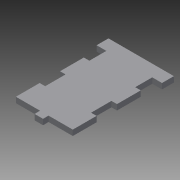
# Autodesk Inventor part: arm-servo
Saved by Autodesk Inventor 2013 (Build 170138000, 138)
## iProperties
Created: 2012-09-08
Part Number: arm-servo
Material: Generic
Document SubType Name: Modeling
Designer: frankenteddy
Density: 1 g/cm^3
Author: frankenteddy
Autodesk Inventor part; units mm, degrees
ref_plane "YZ Plane" through (0, 0, 0) normal (1, 0, 0) x (0, 1, 0)
ref_plane "XZ Plane" through (0, 0, 0) normal (0, 1, 0) x (-1, 0, 0)
ref_plane "XY Plane" through (0, 0, 0) normal (0, 0, 1) x (1, 0, 0)
sketch "Block1" plane through (0, 0, 0) normal (0, 0, 1) x (1, 0, 0)
  circle A0 centre (74.029, 24.2723) radius 1
  line L0 (49.279, 30.4723) -> (71.779, 30.4723)
  line L1 (71.779, 30.4723) -> (71.779, 18.0723)
  line L2 (71.779, 18.0723) -> (49.279, 18.0723)
  line L3 (49.279, 18.0723) -> (49.279, 30.4723)
  line L4 (49.279, 30.4723) -> (44.779, 30.4723)
  line L5 (44.779, 30.4723) -> (44.779, 18.0723)
  line L6 (44.779, 18.0723) -> (49.279, 18.0723)
  line L7 (49.279, 18.0723) -> (49.279, 30.4723)
  line L8 (71.779, 30.4723) -> (76.279, 30.4723)
  line L9 (76.279, 30.4723) -> (76.279, 18.0723)
  line L10 (76.279, 18.0723) -> (71.779, 18.0723)
  line L11 (71.779, 18.0723) -> (71.779, 30.4723)
  line L12 (44.779, 24.2723) -> (76.279, 24.2723) construction
  line L13 (47.029, 30.4723) -> (47.029, 18.0723) construction
  circle A1 centre (47.029, 24.2723) radius 1
  line L14 (74.029, 30.4723) -> (74.029, 18.0723) construction
  point P0 (60.979, 24.0984)
  dimension "d7" = 22.5
  dimension "d8" = 12.4
  dimension "d9" = 4.5
  dimension "d10" = 4.5
  dimension "d11" = 2
  dimension "d12" = 2
  measures "d7" distance of L1.end L2.end
  measures "d8" distance of L0.end L1.end
  measures "d9" distance of L6.end L5.end
  measures "d10" distance of L9.end L10.end
  measures "d11" diameter of A0
  measures "d12" diameter of A1
sketch "Sketch1" plane through (0, 0, 0) normal (0, 0, 1) x (1, 0, 0)
  line L0 (-38.4282, 40.714) -> (0.0718, 40.714)
  line L1 (0.0718, 40.714) -> (0.0718, 33.714)
  line L2 (0.0718, 33.714) -> (-38.4282, 33.714)
  line L3 (-38.4282, 33.714) -> (-38.4282, 40.714)
  line L4 (-92.7646, -8.503) -> (-89.7646, -8.503)
  line L5 (-89.7646, -8.503) -> (-89.7646, -11.753)
  line L6 (-89.7646, -11.753) -> (-92.7646, -11.753)
  line L7 (-92.7646, -11.753) -> (-92.7646, -8.503)
  line L8 (-92.7646, -21.6527) -> (-89.7646, -21.6527)
  line L9 (-89.7646, -21.6527) -> (-89.7646, -21.7527)
  line L10 (-89.7646, -21.7527) -> (-92.7646, -21.7527)
  line L11 (-92.7646, -21.7527) -> (-92.7646, -21.6527)
  line L12 (-32.6782, 33.714) -> (-5.6782, 33.714)
  line L13 (-5.6782, 33.714) -> (-5.6782, -16.286)
  line L14 (-5.6782, -16.286) -> (-32.6782, -16.286)
  line L15 (-32.6782, -16.286) -> (-32.6782, 33.714)
  line L16 (-19.1782, 40.714) -> (-19.1782, 33.714) construction
  line L17 (-19.1782, -16.286) -> (-19.1782, 33.714) construction
  line L18 (-35.9282, 23.714) -> (-32.6782, 23.714)
  line L19 (-32.6782, 23.714) -> (-32.6782, 9.714)
  line L20 (-32.6782, 9.714) -> (-35.9282, 9.714)
  line L21 (-35.9282, 9.714) -> (-35.9282, 23.714)
  line L22 (-2.4282, 23.714) -> (-5.6782, 23.714)
  line L23 (-5.6782, 23.714) -> (-5.6782, 9.714)
  line L24 (-5.6782, 9.714) -> (-2.4282, 9.714)
  line L25 (-2.4282, 9.714) -> (-2.4282, 23.714)
  line L26 (-35.9282, -2.286) -> (-32.6782, -2.286)
  line L27 (-32.6782, -2.286) -> (-32.6782, -16.286)
  line L28 (-32.6782, -16.286) -> (-35.9282, -16.286)
  line L29 (-35.9282, -16.286) -> (-35.9282, -2.286)
  line L30 (-2.4282, -2.286) -> (-5.6782, -2.286)
  line L31 (-5.6782, -2.286) -> (-5.6782, -16.286)
  line L32 (-5.6782, -16.286) -> (-2.4282, -16.286)
  line L33 (-2.4282, -16.286) -> (-2.4282, -2.286)
  line L34 (-21.6782, -16.286) -> (-16.6782, -16.286)
  line L35 (-16.6782, -16.286) -> (-16.6782, -19.536)
  line L36 (-16.6782, -19.536) -> (-21.6782, -19.536)
  line L37 (-21.6782, -19.536) -> (-21.6782, -16.286)
  line L38 (-19.1782, -16.286) -> (-19.1782, -19.536) construction
  point P0 (0, 0)
  dimension "d0" = 3
  dimension "mat" = 3.25
  dimension "d2" = 3
  dimension "d3" = 0.1
  dimension "d4" = 38.5
  dimension "d6" = 7
  dimension "d17" = 27
  dimension "d20" = 50
  dimension "d23" = 3.25
  dimension "d24" = 14
  dimension "d25" = 10
  dimension "d26" = 3.25
  dimension "d27" = 14
  dimension "d28" = 5
  dimension "d29" = 3.25
  constraints: 78 end point, 14 parallel, 9 symmetric about line, 7 perpendicular, 6 collinear, 6 horizontal, 6 midpoint, 1 point on line
  measures "d0" distance of L5.end L7.start
  measures "mat" distance of L5.start L5.end
  measures "d2" distance of L9.end L11.start
  measures "d3" distance of L9.start L9.end
  measures "d4" distance of L1.end L2.end
  measures "d6" distance of L0.end L1.end
  measures "d17" distance of L13.end L14.end
  measures "d20" distance of L12.end L13.end
  measures "d23" distance of L19.end L20.end
  measures "d24" distance of L18.end L19.end
  measures "d25" distance between parallel lines of L18 L2
  measures "d26" distance of L27.end L28.end
  measures "d27" distance of L26.end L27.end
  measures "d28" distance of L35.end L36.end
  measures "d29" distance of L34.end L35.end
extrude "Extrusion2" add sketch "Sketch1" along normal blind 3.25 contours L0 L1 L2 L3 | L2 L13 L14 L15 | L15 L20 L21 L18 | L22 L25 L24 L13 | L15 L28 L29 L26 | L30 L33 L32 L13 | L14 L35 L36 L37
equation "\"d23\" = mat"
equation "\"d26\" = mat"
equation "\"d29\" = mat"
equation "\"d30\" = mat"
body "Solid2"
